Autodesk Inventor part; units mm, degrees
(part 2 of 2)
sketch "スケッチ36" plane through (0, 0, 35) normal (0, 0, 1) x (1, 0, 0)
  arc A0 (-10.4656, -52.9761) -> (-12.7851, -54.4206) centre (-10.8532, -54.9382) ccw projected
  line L0 (-12.7851, -54.4206) -> (-13.3928, -56.6885) projected
  arc A1 (-13.3928, -56.6885) -> (-12.4721, -58.9317) centre (-11.4609, -57.2061) ccw projected
  arc A2 (-10, -63.2456) -> (-12.4721, -58.9317) centre (-15, -63.2456) ccw projected
  line L1 (-10, -63.2456) -> (-10, -131.4702) projected
  arc A3 (-10, -131.4702) -> (-9, -133.2022) centre (-8, -131.4702) ccw projected
  line L2 (-9, -133.2022) -> (-5, -135.5117) projected
  arc A4 (-5, -135.5117) -> (-3, -135.5117) centre (-4, -133.7796) ccw projected
  line L3 (-3, -135.5117) -> (1, -133.2022) projected
  arc A5 (1, -133.2022) -> (2, -131.4702) centre (0, -131.4702) ccw projected
  line L4 (2, -131.4702) -> (2, -126.8514) projected
  arc A6 (2, -126.8514) -> (1, -125.1193) centre (0, -126.8514) ccw projected
  line L5 (1, -125.1193) -> (-3, -122.8099) projected
  arc A7 (-4, -121.0779) -> (-3, -122.8099) centre (-2, -121.0779) ccw projected
  line L6 (-4, -121.0779) -> (-4, -107.2437) projected
  arc A8 (-3, -105.5117) -> (-4, -107.2437) centre (-2, -107.2437) ccw projected
  line L7 (-3, -105.5117) -> (1, -103.2022) projected
  arc A9 (1, -103.2022) -> (2, -101.4702) centre (0, -101.4702) ccw projected
  line L8 (2, -101.4702) -> (2, -96.8514) projected
  arc A10 (2, -96.8514) -> (1, -95.1193) centre (0, -96.8514) ccw projected
  line L9 (1, -95.1193) -> (-3, -92.8099) projected
  arc A11 (-4, -91.0779) -> (-3, -92.8099) centre (-2, -91.0779) ccw projected
  line L10 (-4, -91.0779) -> (-4, -77.2437) projected
  arc A12 (-3, -75.5117) -> (-4, -77.2437) centre (-2, -77.2437) ccw projected
  line L11 (-3, -75.5117) -> (1, -73.2022) projected
  arc A13 (1, -73.2022) -> (2, -71.4702) centre (0, -71.4702) ccw projected
  line L12 (2, -71.4702) -> (2, -66.8514) projected
  arc A14 (2, -66.8514) -> (1, -65.1193) centre (0, -66.8514) ccw projected
  line L13 (1, -65.1193) -> (-3, -62.8099) projected
  arc A15 (-4, -61.0779) -> (-3, -62.8099) centre (-2, -61.0779) ccw projected
  line L14 (-4, -61.0779) -> (-4, -58.3095) projected
  arc A16 (-4, -58.3095) -> (-8.2373, -53.368) centre (-9, -58.3095) ccw projected
  arc A17 (-10.4656, -52.9761) -> (-8.2373, -53.368) centre (0, 0) ccw projected
  line L15 (-1, -130.8928) -> (-4, -132.6249) projected
  line L16 (-4, -132.6249) -> (-7, -130.8928) projected
  line L17 (-7, -130.8928) -> (-7, -127.4287) projected
  line L18 (-7, -127.4287) -> (-4, -125.6967) projected
  line L19 (-4, -125.6967) -> (-1, -127.4287) projected
  line L20 (-1, -127.4287) -> (-1, -130.8928) projected
  line L21 (-4, -102.6249) -> (-7, -100.8928) projected
  line L22 (-7, -100.8928) -> (-7, -97.4287) projected
  line L23 (-7, -97.4287) -> (-4, -95.6967) projected
  line L24 (-4, -95.6967) -> (-1, -97.4287) projected
  line L25 (-1, -97.4287) -> (-1, -100.8928) projected
  line L26 (-1, -100.8928) -> (-4, -102.6249) projected
  line L27 (-4, -65.6967) -> (-1, -67.4287) projected
  line L28 (-1, -67.4287) -> (-1, -70.8928) projected
  line L29 (-1, -70.8928) -> (-4, -72.6249) projected
  line L30 (-4, -72.6249) -> (-7, -70.8928) projected
  line L31 (-7, -70.8928) -> (-7, -67.4287) projected
  line L32 (-7, -67.4287) -> (-4, -65.6967) projected
  arc A18 (60, -32) -> (58, -30) centre (58, -32) ccw projected
  line L33 (58, -30) -> (55.9991, -30) projected
  arc A19 (55.9991, -30) -> (53.9996, -31.9585) centre (55.9991, -32) ccw projected
  arc A20 (53, -33.6491) -> (53.9996, -31.9585) centre (52, -31.9171) ccw projected
  line L34 (53, -33.6491) -> (49, -35.9585) projected
  arc A21 (49, -35.9585) -> (48, -37.6906) centre (50, -37.6906) ccw projected
  line L35 (48, -37.6906) -> (48, -42.3094) projected
  arc A22 (48, -42.3094) -> (49, -44.0415) centre (50, -42.3094) ccw projected
  line L36 (49, -44.0415) -> (53, -46.3509) projected
  arc A23 (54, -48.0829) -> (53, -46.3509) centre (52, -48.0829) ccw projected
  line L37 (54, -48.0829) -> (54, -71.9171) projected
  arc A24 (53, -73.6491) -> (54, -71.9171) centre (52, -71.9171) ccw projected
  line L38 (53, -73.6491) -> (49, -75.9585) projected
  arc A25 (49, -75.9585) -> (48, -77.6906) centre (50, -77.6906) ccw projected
  line L39 (48, -77.6906) -> (48, -82.3094) projected
  arc A26 (48, -82.3094) -> (49, -84.0415) centre (50, -82.3094) ccw projected
  line L40 (49, -84.0415) -> (53, -86.3509) projected
  arc A27 (54, -88.0829) -> (53, -86.3509) centre (52, -88.0829) ccw projected
  line L41 (54, -88.0829) -> (54, -111.9171) projected
  arc A28 (53, -113.6491) -> (54, -111.9171) centre (52, -111.9171) ccw projected
  line L42 (53, -113.6491) -> (49, -115.9585) projected
  arc A29 (49, -115.9585) -> (48, -117.6906) centre (50, -117.6906) ccw projected
  line L43 (48, -117.6906) -> (48, -122.3094) projected
  arc A30 (48, -122.3094) -> (49, -124.0415) centre (50, -122.3094) ccw projected
  line L44 (49, -124.0415) -> (53, -126.3509) projected
  arc A31 (54, -128.0829) -> (53, -126.3509) centre (52, -128.0829) ccw projected
  line L45 (54, -128.0829) -> (54, -151.9171) projected
  arc A32 (53, -153.6491) -> (54, -151.9171) centre (52, -151.9171) ccw projected
  line L46 (53, -153.6491) -> (49, -155.9585) projected
  arc A33 (49, -155.9585) -> (48, -157.6906) centre (50, -157.6906) ccw projected
  line L47 (48, -157.6906) -> (48, -162.3094) projected
  arc A34 (48, -162.3094) -> (49, -164.0415) centre (50, -162.3094) ccw projected
  line L48 (49, -164.0415) -> (53, -166.3509) projected
  arc A35 (53, -166.3509) -> (55, -166.3509) centre (54, -164.6188) ccw projected
  line L49 (55, -166.3509) -> (59, -164.0415) projected
  arc A36 (59, -164.0415) -> (60, -162.3094) centre (58, -162.3094) ccw projected
  line L50 (60, -162.3094) -> (60, -32) projected
  line L51 (51, -38.2679) -> (54, -36.5359) projected
  line L52 (54, -36.5359) -> (57, -38.2679) projected
  line L53 (57, -38.2679) -> (57, -41.7321) projected
  line L54 (57, -41.7321) -> (54, -43.4641) projected
  line L55 (54, -43.4641) -> (51, -41.7321) projected
  line L56 (51, -41.7321) -> (51, -38.2679) projected
  line L57 (51, -158.2679) -> (54, -156.5359) projected
  line L58 (54, -156.5359) -> (57, -158.2679) projected
  line L59 (57, -158.2679) -> (57, -161.7321) projected
  line L60 (57, -161.7321) -> (54, -163.4641) projected
  line L61 (54, -163.4641) -> (51, -161.7321) projected
  line L62 (51, -161.7321) -> (51, -158.2679) projected
  line L63 (51, -78.2679) -> (54, -76.5359) projected
  line L64 (54, -76.5359) -> (57, -78.2679) projected
  line L65 (57, -78.2679) -> (57, -81.7321) projected
  line L66 (57, -81.7321) -> (54, -83.4641) projected
  line L67 (54, -83.4641) -> (51, -81.7321) projected
  line L68 (51, -81.7321) -> (51, -78.2679) projected
  line L69 (51, -118.2679) -> (54, -116.5359) projected
  line L70 (54, -116.5359) -> (57, -118.2679) projected
  line L71 (57, -118.2679) -> (57, -121.7321) projected
  line L72 (57, -121.7321) -> (54, -123.4641) projected
  line L73 (54, -123.4641) -> (51, -121.7321) projected
  line L74 (51, -121.7321) -> (51, -118.2679) projected
  line L75 (-1.1, -67.4865) -> (-4, -65.8122)
  line L76 (-4, -65.8122) -> (-6.9, -67.4865)
  line L77 (-6.9, -67.4865) -> (-6.9, -70.8351)
  line L78 (-6.9, -70.8351) -> (-4, -72.5094)
  line L79 (-4, -72.5094) -> (-1.1, -70.8351)
  line L80 (-1.1, -70.8351) -> (-1.1, -67.4865)
  line L81 (-4, -95.8122) -> (-6.9, -97.4865)
  line L82 (-6.9, -97.4865) -> (-6.9, -100.8351)
  line L83 (-6.9, -100.8351) -> (-4, -102.5094)
  line L84 (-4, -102.5094) -> (-1.1, -100.8351)
  line L85 (-1.1, -100.8351) -> (-1.1, -97.4865)
  line L86 (-1.1, -97.4865) -> (-4, -95.8122)
  line L87 (-4, -125.8122) -> (-6.9, -127.4865)
  line L88 (-6.9, -127.4865) -> (-6.9, -130.8351)
  line L89 (-6.9, -130.8351) -> (-4, -132.5094)
  line L90 (-4, -132.5094) -> (-1.1, -130.8351)
  line L91 (-1.1, -130.8351) -> (-1.1, -127.4865)
  line L92 (-1.1, -127.4865) -> (-4, -125.8122)
  line L93 (54, -36.6514) -> (51.1, -38.3257)
  line L94 (51.1, -38.3257) -> (51.1, -41.6743)
  line L95 (51.1, -41.6743) -> (54, -43.3486)
  line L96 (54, -43.3486) -> (56.9, -41.6743)
  line L97 (56.9, -41.6743) -> (56.9, -38.3257)
  line L98 (56.9, -38.3257) -> (54, -36.6514)
  line L99 (54, -76.6514) -> (51.1, -78.3257)
  line L100 (51.1, -78.3257) -> (51.1, -81.6743)
  line L101 (51.1, -81.6743) -> (54, -83.3486)
  line L102 (54, -83.3486) -> (56.9, -81.6743)
  line L103 (56.9, -81.6743) -> (56.9, -78.3257)
  line L104 (56.9, -78.3257) -> (54, -76.6514)
  line L105 (54, -116.6514) -> (51.1, -118.3257)
  line L106 (51.1, -118.3257) -> (51.1, -121.6743)
  line L107 (51.1, -121.6743) -> (54, -123.3486)
  line L108 (54, -123.3486) -> (56.9, -121.6743)
  line L109 (56.9, -121.6743) -> (56.9, -118.3257)
  line L110 (56.9, -118.3257) -> (54, -116.6514)
  line L111 (54, -156.6514) -> (51.1, -158.3257)
  line L112 (51.1, -158.3257) -> (51.1, -161.6743)
  line L113 (51.1, -161.6743) -> (54, -163.3486)
  line L114 (54, -163.3486) -> (56.9, -161.6743)
  line L115 (56.9, -161.6743) -> (56.9, -158.3257)
  line L116 (56.9, -158.3257) -> (54, -156.6514)
  point P0 (-1.1, -129.1608)
  dimension "d503" = 0.1
  dimension "d504" = 0.1
  dimension "d505" = 0.1
  dimension "d506" = 0.1
  dimension "d507" = 0.1
  dimension "d508" = 0.1
  dimension "d509" = 0.1
  constraints: 84 end point, 1 midpoint, 35 other
  measures "d503" distance between parallel lines of L28 L80
  measures "d504" distance between parallel lines of L25 L85
  measures "d505" distance from line of L20 point (-1.1, -129.161)
  measures "d506" distance between parallel lines of L62 L112
  measures "d507" distance between parallel lines of L74 L106
  measures "d508" distance between parallel lines of L68 L100
  measures "d509" distance between parallel lines of L56 L94
extrude "押し出し21" add sketch "スケッチ36" against normal blind 30 contours L15 L16 L17 L18 L19 L20 | L21 L22 L23 L24 L25 L26 | L27 L28 L29 L30 L31 L32 | L51 L52 L53 L54 L55 L56 | L57 L58 L59 L60 L61 L62 | L63 L64 L65 L66 L67 L68 | L69 L70 L71 L72 L73 L74
equation "\"d25\" = d24"
equation "\"d90\" = d89"
